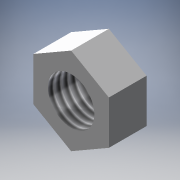
# Autodesk Inventor part: Nut_Normal
Saved by Autodesk Inventor 2016 (Build 200138000, 138)
## iProperties
Created: 2016-04-23
Part Number: Nut_Normal
Material: Generic
Document SubType Name: Modeling
Designer: 3DPrinterUser
Density: 1 g/cm^3
Appearance: Aluminum - Flat
Author: 3DPrinterUser
Autodesk Inventor part; units mm, degrees
ref_plane "YZ Plane" through (0, 0, 0) normal (1, 0, 0) x (0, 1, 0)
ref_plane "XZ Plane" through (0, 0, 0) normal (0, 1, 0) x (-1, 0, 0)
ref_plane "XY Plane" through (0, 0, 0) normal (0, 0, 1) x (1, 0, 0)
sketch "Sketch1" plane through (0, 0, 0) normal (0, 1, 0) x (-1, 0, 0)
  line L0 (0, -7.5056) -> (-6.5, -3.7528)
  line L1 (-6.5, -3.7528) -> (-6.5, 3.7528)
  line L2 (-6.5, 3.7528) -> (0, 7.5056)
  line L3 (0, 7.5056) -> (6.5, 3.7528)
  line L4 (6.5, 3.7528) -> (6.5, -3.7528)
  line L5 (6.5, -3.7528) -> (0, -7.5056)
  circle A0 centre (0, 0) radius 4
  dimension "d0" = 13
  dimension "d1" = 8
  constraints: 12 end point, 2 coincident, 1 centre point, 13 other
  measures "d0" distance between parallel lines of L5 L2
  measures "d1" diameter of A0
extrude "Extrusion1" add sketch "Sketch1" along normal blind 6.5
thread "Thread1" size "M8x1.25" class "6H" standard "ANSI Metric M Profile" full length
body "Solid1"
